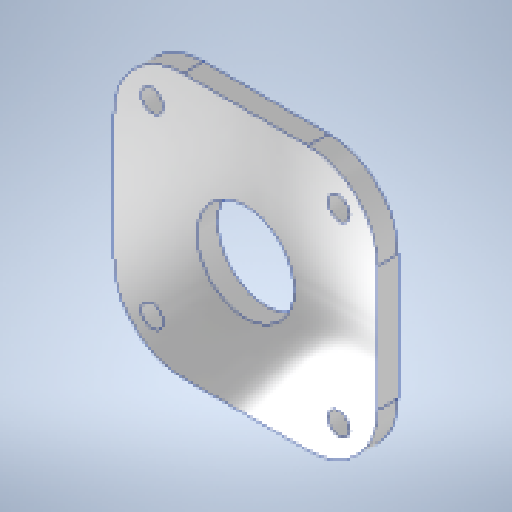
# Autodesk Inventor part: hand1_part3
Saved by Autodesk Inventor 2024 (Build 280153000, 153)
## iProperties
Created: 2025-02-21
Part Number: hand1_part3
Material: アルミニウム 6061
Document SubType Name: Modeling
Designer: tanoue_kota
Density: 2.7 g/cm^3
Appearance: アルミニウム - フラット
Author: tanoue_kota
Autodesk Inventor part; units mm, degrees
ref_plane "YZ Plane" through (0, 0, 0) normal (1, 0, 0) x (0, 1, 0)
ref_plane "XZ Plane" through (0, 0, 0) normal (0, 1, 0) x (-1, 0, 0)
ref_plane "XY Plane" through (0, 0, 0) normal (0, 0, 1) x (1, 0, 0)
sketch "スケッチ1" plane through (0, 0, 0) normal (0, 0, 1) x (1, 0, 0)
  circle A0 centre (0, 0) radius 19
  line L0 (-19, 19) -> (19, 19)
  line L1 (19, 19) -> (19, -19)
  line L2 (19, -19) -> (-19, -19)
  line L3 (-19, -19) -> (-19, 19)
  dimension "d0" = 38
  constraints: 8 end point, 4 tangent, 2 parallel, 1 centre point, 1 coincident, 1 horizontal, 1 perpendicular
  measures "d0" diameter of A0
extrude "押し出し1" add sketch "スケッチ1" along normal blind 3
sketch "スケッチ2" plane through (0, 0, 3) normal (0, 0, 1) x (1, 0, 0)
  circle A0 centre (0, 0) radius 7
  dimension "d3" = 14
  constraints: 1 centre point, 1 coincident
  measures "d3" diameter of A0
extrude "押し出し2" cut sketch "スケッチ2" against normal blind 3
sketch "スケッチ3" plane through (0, 0, 3) normal (0, 0, 1) x (1, 0, 0)
  circle A0 centre (0, 0) radius 19
  line L0 (0, 0) -> (-13.435, 13.435)
  line L1 (0, 0) -> (0, 19)
  point P0 (-13.435, -13.435)
  point P1 (13.435, -13.435)
  point P2 (13.435, 13.435)
  dimension "d6" = 38
  dimension "d7" = 45
  dimension "d10" = 360
  constraints: 4 end point, 2 point on circle, 1 centre point, 1 coincident, 1 vertical, 5 other
  measures "d6" diameter of A0
  measures "d7" angle of L1 L0
hole "穴1" at (-13.435, 13.435, 3) at (-13.435, -13.435, 3) at (13.435, -13.435, 3) at (13.435, 13.435, 3) direction (0, 0, -1) diameter 3.2 end through all
fillet "フィレット1" radius 10 4 edges at (-19, 19, 1.5) (19, 19, 1.5) (19, -19, 1.5) (-19, -19, 1.5)
